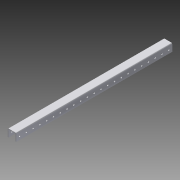
# Autodesk Inventor part: CornerChannel
Saved by Autodesk Inventor 2015 (Build 190159000, 159)
## iProperties
Created: 2015-01-26
Part Number: CornerChannel
Material: Aluminum 6061
Document SubType Name: Modeling
Designer: Andrew
Density: 2.7 g/cm^3
Appearance: Aluminum - Flat
SupportLength: 23.000 in
Author: Andrew
Autodesk Inventor part; units mm, degrees
ref_plane "YZ Plane" through (0, 0, 0) normal (1, 0, 0) x (0, 1, 0)
ref_plane "XZ Plane" through (0, 0, 0) normal (0, 1, 0) x (-1, 0, 0)
ref_plane "XY Plane" through (0, 0, 0) normal (0, 0, 1) x (1, 0, 0)
sketch "Sketch1" plane through (0, 0, 0) normal (0, 0, 1) x (1, 0, 0)
  line L0 (-15.875, 0) -> (-12.7, 0)
  line L1 (-12.7, 0) -> (-12.7, 22.352)
  line L2 (-9.525, 25.527) -> (9.525, 25.527)
  line L3 (12.7, 22.352) -> (12.7, 0)
  line L4 (12.7, 0) -> (15.875, 0)
  line L5 (15.875, 0) -> (15.875, 25.527)
  line L6 (12.7, 28.702) -> (-12.7, 28.702)
  line L7 (-15.875, 25.527) -> (-15.875, 0)
  arc A0 (-9.525, 25.527) -> (-12.7, 22.352) centre (-9.525, 22.352) ccw
  arc A1 (12.7, 22.352) -> (9.525, 25.527) centre (9.525, 22.352) ccw
  arc A2 (-12.7, 28.702) -> (-15.875, 25.527) centre (-12.7, 25.527) ccw
  arc A3 (15.875, 25.527) -> (12.7, 28.702) centre (12.7, 25.527) ccw
  line L8 (0, 35.2315) -> (0, -5.8719) projected
  point P0 (0, 0)
  dimension "d0" = 28.702
  dimension "d1" = 31.75
  dimension "d2" = 3.175
  dimension "d3" = 3.175
  dimension "d4" = 3.175
  constraints: 16 end point, 8 point on circle, 8 tangent, 6 perpendicular, 4 centre point, 3 equal radius, 3 point on line, 1 horizontal, 2 other
  measures "d0" distance between parallel lines of L4 L6
  measures "d1" distance between parallel lines of L5 L7
  measures "d2" distance between parallel lines of L5 L3
  measures "d3" distance between parallel lines of L2 L6
  measures "d4" radius of A0
extrude "Extrusion1" add sketch "Sketch1" along normal mid plane 584.2
sketch "Sketch4" plane through (15.875, 0, 292.1) normal (1, 0, 0) x (0, 0, -1)
  line L0 (292.1, -5.7404) -> (292.1, 34.4424) construction
  line L1 (-116.84, 0) -> (701.04, 0) construction
  circle A0 centre (292.1, 12.7) radius 3.175
  point P0 (292.1, 0)
  dimension "d34" = 12.7
  dimension "d35" = 0
  dimension "d36" = 6.35
  constraints: 1 centre point
  measures "d34" distance from line of L1 A0.centre
  measures "d35" distance from line of L0 A0.centre
  measures "d36" diameter of A0
extrude "Extrusion4" cut sketch "Sketch4" against normal up to surface (31.75 mm away)
pattern_linear "Rectangular Pattern3" count 15 spacing 25.4 along (0, 0, 1) count 15 spacing 25.4 along (0, 0, -1) of "Extrusion4"
equation "\"d5\" = SupportLength"
equation "\"SupportLength\" = 584.2"
body "Solid1"
